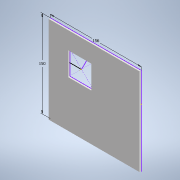
# Autodesk Inventor part: box bottom
Saved by Autodesk Inventor 2020 (Build 240168000, 168)
## iProperties
Created: 2020-12-15
Part Number: box bottom
Material: Generic
Document SubType Name: Modeling
Designer: moham
Density: 1 g/cm^3
Appearance: Default
Author: moham
Autodesk Inventor part; units mm, degrees
ref_plane "YZ Plane" through (0, 0, 0) normal (1, 0, 0) x (0, 1, 0)
ref_plane "XZ Plane" through (0, 0, 0) normal (0, 1, 0) x (-1, 0, 0)
ref_plane "XY Plane" through (0, 0, 0) normal (0, 0, 1) x (1, 0, 0)
sketch "Sketch1" plane through (0, 0, 0) normal (0, 0, 1) x (1, 0, 0)
  line L0 (-53, 50) -> (103, 50)
  line L1 (-53, 50) -> (-53, -100)
  line L2 (-53, -100) -> (103, -100)
  line L3 (103, -100) -> (103, 50)
  line L4 (0, 0) -> (-53, 0)
  line L5 (0, 0) -> (25, 50)
  line L6 (103, 50) -> (23, 50)
  line L7 (-20, -20) -> (20, -20)
  line L8 (20, -20) -> (20, 20)
  line L9 (20, 20) -> (-20, 20)
  line L10 (-20, 20) -> (-20, -20)
  line L11 (-20, -20) -> (20, 20) construction
  line L12 (20, -20) -> (-20, 20) construction
  dimension "d0" = 156
  dimension "d1" = 150
  constraints: 26 end point, 4 perpendicular, 3 midpoint, 2 horizontal, 2 parallel, 2 point on line, 1 vertical
  measures "d0" distance of L0.start L0.end
  measures "d1" distance of L0.start L1.end
sketch "Sketch2" plane through (0, 0, 0) normal (0, 0, 1) x (1, 0, 0)
  point P0 (0, 0)
extrude "Extrusion1" add sketch "Sketch1" along normal blind 3
sketch "Sketch3" plane through (103, -100, 0) normal (1, 0, 0) x (0, 0, -1)
  point P0 (0, 100)
sketch "Sketch4" plane through (0, 0, 0) normal (0, 0, 1) x (1, 0, 0)
  point P0 (0, 0)
extrude "Extrusion3" cut sketch "Sketch1" along normal blind 10 contours L10 L9 L5 L4 | L4 L5 L9 L8 L7 L10
body "Solid1"
